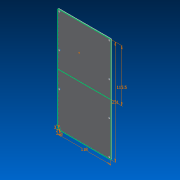
# Autodesk Inventor part: case lid
Saved by Autodesk Inventor 2015 (Build 190159000, 159)
## iProperties
Created: 2017-03-22
Part Number: case lid
Material: Generic
Document SubType Name: Modeling
Designer: ZigZagJoe
Density: 1 g/cm^3
Appearance: Default
Author: ZigZagJoe
Autodesk Inventor part; units mm, degrees
ref_plane "YZ Plane" through (0, 0, 0) normal (1, 0, 0) x (0, 1, 0)
ref_plane "XZ Plane" through (0, 0, 0) normal (0, 1, 0) x (-1, 0, 0)
ref_plane "XY Plane" through (0, 0, 0) normal (0, 0, 1) x (1, 0, 0)
sketch "Sketch1" plane through (0, 0, 0) normal (0, 1, 0) x (-1, 0, 0)
  line L0 (48.0552, 60.6643) -> (-69.9448, 60.6643)
  line L1 (-69.9448, 60.6643) -> (-69.9448, -170.3357)
  line L2 (-69.9448, -170.3357) -> (48.0552, -170.3357)
  line L3 (48.0552, -170.3357) -> (48.0552, 60.6643)
  line L4 (48.0552, -54.8357) -> (-69.9448, -54.8357)
  circle A0 centre (44.5552, -166.8357) radius 1.5
  point P0 (0, 0)
  dimension "d0" = 118
  dimension "d1" = 231
  dimension "d2" = 115.5
  dimension "d3" = 3
  dimension "d4" = 3.5
  dimension "d5" = 3.5
  constraints: 10 end point, 2 midpoint, 2 parallel, 2 perpendicular, 1 centre point, 1 horizontal
  measures "d0" distance of L2.end L1.end
  measures "d1" distance of L1.end L0.end
  measures "d2" distance between parallel lines of L4 L0
  measures "d3" diameter of A0
  measures "d4" distance from line of L2 A0.centre
  measures "d5" distance from line of L3 A0.centre
extrude "Base" add sketch "Sketch1" along normal blind 2 contours L3 L4 L1 L0 | L3 L2 L1 L4 | A0
extrude "Screw Hole" cut sketch "Sketch1" along normal blind 3 contours A0
pattern_linear "Screw Hole Pattern" count 4 spacing 74.666 along (0, 0, 1) count 2 spacing 111 along (1, 0, 0) of "Screw Hole"
fillet "Corner Fillet" radius 1.2 4 edges at (69.9448, 1, 60.6643) (-48.0552, 1, 60.6643) (69.9448, 1, -170.3357) (-48.0552, 1, -170.3357)
extrude "Sectioning Cut (rear only)" [suppressed]
extrude "Sectioning Cut (front only)" [suppressed]
body "Solid1"
